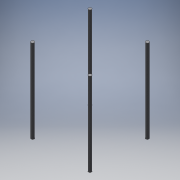
# Autodesk Inventor part: TrnlloSinFin
Saved by Autodesk Inventor 2017 (Build 210142000, 142)
## iProperties
Part Number: TrnlloSinFin
Material: Genérico
Document SubType Name: Modeling
Designer: Leonardo
Density: 1 g/cm^3
Appearance: Valor por defecto
Author: Leonardo
Autodesk Inventor part; units mm, degrees
ref_plane "YZ Plane" through (0, 0, 0) normal (1, 0, 0) x (0, 1, 0)
ref_plane "XZ Plane" through (0, 0, 0) normal (0, 1, 0) x (-1, 0, 0)
ref_plane "XY Plane" through (0, 0, 0) normal (0, 0, 1) x (1, 0, 0)
sketch "Boceto1" plane through (0, 0, 0) normal (0, 0, 1) x (1, 0, 0)
  circle A0 centre (58.5, 58.5) radius 3.175 projected
  circle A1 centre (58.5, -58.5) radius 3.175 projected
  circle A2 centre (-58.5, -58.5) radius 3.175 projected
  circle A3 centre (-58.5, 58.5) radius 3.175 projected
  point P0 (0, 0)
extrude "Extrusión1" add sketch "Boceto1" along normal blind 170
thread "Rosca1" size "M7x1" class "6g" standard "ANSI Metric M Profile" full length
thread "Rosca2" size "M7x1" class "6g" standard "ANSI Metric M Profile" full length
thread "Rosca3" size "M7x1" class "6g" standard "ANSI Metric M Profile" full length
thread "Rosca4" size "M7x1" class "6g" standard "ANSI Metric M Profile" full length
